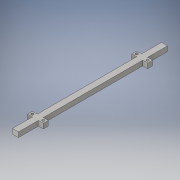
# Autodesk Inventor part: Rack Bottom
Saved by Autodesk Inventor 2016 (Build 200138000, 138)
## iProperties
Created: 2016-04-15
Part Number: Rack Bottom
Material: Generic
Document SubType Name: Modeling
Designer: Andrea
Density: 1 g/cm^3
Appearance: Default
Author: Andrea
Autodesk Inventor part; units mm, degrees
ref_plane "YZ Plane" through (0, 0, 0) normal (1, 0, 0) x (0, 1, 0)
ref_plane "XZ Plane" through (0, 0, 0) normal (0, 1, 0) x (-1, 0, 0)
ref_plane "XY Plane" through (0, 0, 0) normal (0, 0, 1) x (1, 0, 0)
sketch "Sketch1" plane through (0, 0, 0) normal (0, 1, 0) x (-1, 0, 0)
  line L0 (-7.62, 190.5) -> (7.62, 190.5)
  line L1 (7.62, 190.5) -> (7.62, -190.5)
  line L2 (7.62, -190.5) -> (-7.62, -190.5)
  line L3 (-7.62, -190.5) -> (-7.62, 190.5)
  line L4 (-7.62, 190.5) -> (7.62, -190.5) construction
  line L5 (7.62, 190.5) -> (-7.62, -190.5) construction
  point P0 (0, 0)
  dimension "d0" = 15.24
  dimension "d1" = 381
  constraints: 12 end point, 2 midpoint, 2 parallel, 1 horizontal, 1 perpendicular
  measures "d0" distance of L1.end L2.end
  measures "d1" distance of L0.end L1.end
extrude "Extrusion1" add sketch "Sketch1" along normal blind 12.7
sketch "Sketch2" plane through (0, 12.7, 0) normal (0, 1, 0) x (1, 0, 0)
  line L0 (-7.62, 190.5) -> (-7.62, -190.5) projected
  line L1 (-7.62, -139.7) -> (-20.32, -139.7)
  line L2 (-20.32, -139.7) -> (-20.32, -127)
  line L3 (-20.32, -127) -> (-7.62, -127)
  line L4 (-7.62, -127) -> (-7.62, -139.7)
  circle A0 centre (-13.97, -133.35) radius 3.175
  point P0 (0, 0)
  dimension "d4" = 12.7
  dimension "d5" = 12.7
  dimension "d6" = 127
  dimension "d7" = 6.35
  dimension "d8" = 6.35
  dimension "d9" = 6.35
  constraints: 8 end point, 2 parallel, 1 centre point, 1 horizontal, 1 perpendicular, 1 point on line
  measures "d4" distance of L2.end L3.end
  measures "d5" distance of L1.end L2.end
  measures "d6" vertical distance of L3.end point (0, 0)
  measures "d7" diameter of A0
  measures "d8" distance from line of A0.centre L0
  measures "d9" distance from line of A0.centre L1
extrude "Extrusion2" add sketch "Sketch2" against normal up to surface (12.7 mm away)
mirror "Mirror1" about plane through (0, 0, 0) normal (1, 0, 0) of "Extrusion2"
mirror "Mirror2" about plane through (0, 0, 0) normal (0, 0, 1) of "Extrusion2", "Mirror1"
equation "\"d8\" = 0.5 * d4"
equation "\"d9\" = 0.5 * d5"
body "Solid1"
